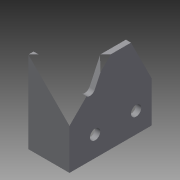
# Autodesk Inventor part: front tab 2x2
Saved by Autodesk Inventor 2015 (Build 190159000, 159)
## iProperties
Created: 2015-02-22
Part Number: front tab 2x2
Material: Generic
Document SubType Name: Modeling
Designer: Jarod
Density: 1 g/cm^3
Appearance: Default
Author: Jarod
Autodesk Inventor part; units mm, degrees
ref_plane "YZ Plane" through (0, 0, 0) normal (1, 0, 0) x (0, 1, 0)
ref_plane "XZ Plane" through (0, 0, 0) normal (0, 1, 0) x (-1, 0, 0)
ref_plane "XY Plane" through (0, 0, 0) normal (0, 0, 1) x (1, 0, 0)
sketch "Sketch1" plane through (0, 0, 0) normal (0, 1, 0) x (-1, 0, 0)
  line L0 (0, 0) -> (50.8, 0)
  line L1 (50.8, 0) -> (50.8, -3.175)
  line L2 (50.8, -3.175) -> (0, -3.175)
  line L3 (0, -3.175) -> (0, 0)
  line L4 (0, 0) -> (3.175, 0)
  line L5 (3.175, 0) -> (3.175, -50.8)
  line L6 (3.175, -50.8) -> (0, -50.8)
  line L7 (0, -50.8) -> (0, 0)
  dimension "d0" = 50.8
  dimension "d1" = 3.175
  dimension "d2" = 3.175
  dimension "d3" = 50.8
  constraints: 16 end point, 4 parallel, 2 horizontal, 2 perpendicular
  measures "d0" distance of L1.end L2.end
  measures "d1" distance of L0.end L1.end
  measures "d2" distance of L5.end L6.end
  measures "d3" distance of L4.end L5.end
extrude "Extrusion1" add sketch "Sketch1" along normal blind 50.8
sketch "Sketch2" plane through (-50.8, 0, 0) normal (0, 0, 1) x (1, 0, 0)
  line L0 (0, 50.8) -> (25.4, 50.8)
  line L1 (25.4, 50.8) -> (25.4, 0)
  line L2 (25.4, 0) -> (0, 0)
  line L3 (0, 0) -> (0, 50.8)
  point P0 (50.8, 0)
  dimension "d6" = 25.4
  dimension "d7" = 50.8
  constraints: 8 end point, 2 parallel, 1 horizontal, 1 perpendicular
  measures "d6" distance of L1.end L2.end
  measures "d7" distance of L0.end L1.end
extrude "Extrusion2" cut sketch "Sketch2" against normal blind 50.8
sketch "Sketch3" plane through (0, 0, 0) normal (1, 0, 0) x (0, 0, -1)
  line L0 (0, 50.8) -> (50.8, 50.8) projected
  line L1 (0, 0) -> (0, 50.8) projected
  line L2 (0, 0) -> (50.8, 0) projected
  line L3 (50.8, 0) -> (50.8, 50.8) projected
  line L4 (3.175, 0) -> (3.175, 50.8) projected
  line L5 (0, 0) -> (3.175, 0) projected
  line L6 (0, 50.8) -> (0, 0) projected
  line L7 (3.175, 50.8) -> (0, 50.8) projected
  circle A0 centre (12.7, 38.1) radius 3.175 construction
  line L8 (3.175, 50.8) -> (9.8303, 36.7415) construction
  line L9 (0, 50.8) -> (50.8, 50.8) construction
  line L10 (22.225, 50.8) -> (15.5697, 36.7415) construction
  line L11 (3.175, 50.8) -> (9.8303, 36.7415)
  line L12 (22.225, 50.8) -> (15.5697, 36.7415)
  arc A1 (9.8303, 36.7415) -> (15.5697, 36.7415) centre (12.7, 38.1) ccw
  line L13 (3.175, 50.8) -> (22.225, 50.8)
  dimension "d10" = 6.35
  dimension "d11" = 19.05
  dimension "d12" = 9.525
  dimension "d13" = 12.7
  constraints: 10 end point, 6 tangent, 4 point on circle, 3 collinear, 2 centre point, 1 point on line
  measures "d10" diameter of A0
  measures "d11" distance of L10.start L4.end
  measures "d12" distance from line of L4 A0.centre
  measures "d13" distance from line of L0 A0.centre
extrude "Extrusion3" cut sketch "Sketch3" against normal blind 50.8 contours L0 L12 A1 L11
sketch "Sketch4" plane through (0, 0, 0) normal (1, 0, 0) x (0, 0, -1)
  line L0 (50.8, 50.8) -> (38.1, 50.8)
  line L1 (22.225, 50.8) -> (50.8, 50.8) projected
  line L2 (50.8, 50.8) -> (50.8, 25.4)
  line L3 (50.8, 0) -> (50.8, 50.8) projected
  line L4 (50.8, 25.4) -> (38.1, 50.8)
  point P0 (0, 0)
  dimension "d16" = 12.7
  dimension "d17" = 25.4
  constraints: 6 end point, 1 midpoint, 1 point on line
  measures "d16" distance of L0.start L0.end
  measures "d17" distance of L0.start L2.end
extrude "Extrusion4" cut sketch "Sketch4" against normal blind 50.8
sketch "Sketch5" plane through (0, 0, 0) normal (1, 0, 0) x (0, 0, -1)
  line L0 (0, 0) -> (0, 50.8) projected
  line L1 (0, 0) -> (50.8, 0) projected
  line L2 (50.8, 0) -> (50.8, 25.4) projected
  point P0 (15.875, 12.7)
  point P1 (41.275, 12.7)
  dimension "d20" = 15.875
  dimension "d21" = 12.7
  dimension "d22" = 12.7
  dimension "d23" = 9.525
  measures "d20" distance from line of L0 point (15.875, 12.7)
  measures "d21" distance from line of L1 point (15.875, 12.7)
  measures "d22" distance from line of L1 point (41.275, 12.7)
  measures "d23" distance from line of L2 point (41.275, 12.7)
hole "Hole1" at (0, 12.7, -15.875) at (0, 12.7, -41.275) direction (-1, 0, 0) diameter 6.35 end through all
body "Solid1"
